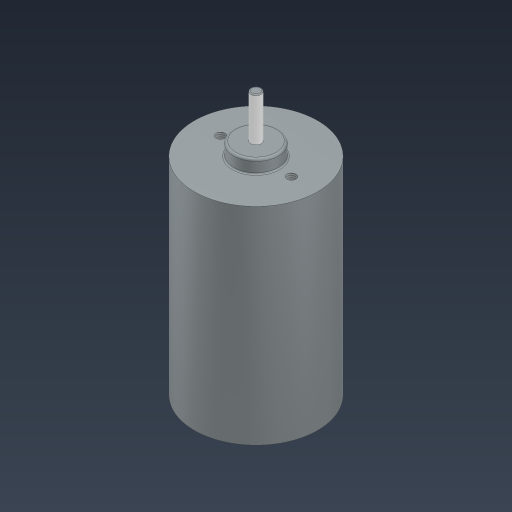
# Autodesk Inventor part: RS395
Saved by Autodesk Inventor 2023 (Build 270158000, 158)
## iProperties
Created: 2025-03-29
Part Number: RS395
Material: Generic
Document SubType Name: Modeling
Designer: szymo
Density: 3.59791 g/cm^3
Appearance: Zinc(1)
Mass: 114.3 g
Surface Area: 60.0998 cm^2
Volume: 31.7685 cm^3
Author: szymo
Autodesk Inventor part; units mm, degrees
ref_plane "YZ Plane" through (0, 0, 0) normal (1, 0, 0) x (0, 1, 0)
ref_plane "XZ Plane" through (0, 0, 0) normal (0, 1, 0) x (-1, 0, 0)
ref_plane "XY Plane" through (0, 0, 0) normal (0, 0, 1) x (1, 0, 0)
sketch "Sketch1" plane through (0, 0, 0) normal (0, 1, 0) x (-1, 0, 0)
  circle A0 centre (0, 0) radius 13.85
  circle A1 centre (0, 0) radius 5
  dimension "d0" = 27.7
  dimension "d3" = 10
  constraints: 2 centre point, 2 coincident
  measures "d0" diameter of A0
  measures "d3" diameter of A1
extrude "Extrusion1" add sketch "Sketch1" along normal blind 46.5 contours A0 | A1
extrude "Extrusion2" add sketch "Sketch1" against normal blind 5.2 contours A1
sketch "Sketch2" plane through (0, 46.5, 0) normal (0, 1, 0) x (1, 0, 0)
  circle A0 centre (0, 0) radius 5
  circle A1 centre (0, 0) radius 1.15
  dimension "d6" = 10
  dimension "d7" = 2.3
  constraints: 2 centre point, 2 coincident
  measures "d6" diameter of A0
  measures "d7" diameter of A1
extrude "Extrusion3" add sketch "Sketch2" along normal blind 3
extrude "Extrusion4" add sketch "Sketch2" along normal blind 12.8 contours A1
ref_plane "Work Plane1" through (0, 41.5, 0) normal (0, 1, 0) x (1, 0, 0)
sketch "Sketch4" plane through (0, 41.5, 0) normal (0, 1, 0) x (1, 0, 0)
  circle A0 centre (0, 0) radius 15.05
  circle A1 centre (0, 0) radius 13.85 projected
  circle A2 centre (0, 0) radius 5 projected
  dimension "d13" = 30.1
  constraints: 1 centre point, 1 coincident
  measures "d13" diameter of A0
extrude "Extrusion5" [suppressed]
sketch "Sketch5" plane through (0, 46.5, 0) normal (0, 1, 0) x (1, 0, 0)
  circle A0 centre (0, 0) radius 1.15 construction
  circle A1 centre (0, 0) radius 6.8 construction
  circle A2 centre (0, 0) radius 13.85 construction
  circle A3 centre (0, 0) radius 9.15 construction
  circle A4 centre (7.975, 0) radius 1.175
  circle A5 centre (-7.975, 0) radius 1.175
  line L0 (0, 0) -> (7.975, 0) construction
  line L1 (0, 0) -> (-7.975, 0) construction
  dimension "d16" = 13.6
  dimension "d17" = 4.7
  constraints: 6 coincident, 4 centre point, 4 end point, 4 tangent, 2 horizontal
  measures "d16" diameter of A1
  measures "d17" radial gap between concentric circles of A2 A3
hole "Hole1" at (-7.975, 46.5, 0) at (7.975, 46.5, 0) direction (0, -1, 0) diameter 2.013 depth 4 thread size "M2.5x0.45" class "6H" standard "ISO Metric profile"
sketch "Sketch6" plane through (0, 0, 0) normal (1, 0, 0) x (0, 1, 0)
  line L0 (-5.2, 5) -> (-5.2, -5) projected
  line L1 (0, -5) -> (0, 5) projected
  line L2 (0, 0) -> (-6.1046, 0)
  line L3 (0, 5) -> (-5.2, 5) projected
  line L4 (-3.3, 5) -> (-3.3, 3.5)
  line L5 (-3.3, 3.5) -> (-4.3, 3.5)
  line L6 (-4.3, 3.5) -> (-4.3, 1.15)
  line L7 (-4.3, 1.15) -> (-5.2, 1.15)
  line L8 (-5.2, 5) -> (-5.2, -5) projected
  point P0 (-5.2, 0)
  dimension "d25" = 0.9
  dimension "d26" = 1.15
  dimension "d27" = 1
  dimension "d28" = 3.5
  constraints: 10 end point, 3 perpendicular, 2 point on line, 1 horizontal, 1 parallel
  measures "d25" distance of L6.end L7.end
  measures "d26" distance between parallel lines of L2 L7
  measures "d27" distance of L4.end L5.end
  measures "d28" distance between parallel lines of L2 L5
revolve "Revolution1" cut sketch "Sketch6" angle 360 about axis through (0, 0, 0) along (0, -1, 0) contours L3 L4 L5 L6 L7 L0
fillet "Fillet1" radius 0.2 1 edges at (0, -5.2, -1.15)
fillet "Fillet3" radius 1 1 edges at (5, 0, 0)
chamfer "Chamfer1" distance 0.4 angle 45 1 edges at (0, -3.3, -3.5)
fillet "Fillet4" radius 0.2 1 edges at (0, -4.3, -3.5)
fillet "Fillet5" radius 0.5 2 edges at (0, -3.3, -3.9) (0, -3.7, -3.5)
fillet "Fillet6" radius 0.2 1 edges at (-1.15, 59.3, 0)
fillet "Fillet7" radius 0.5 1 edges at (-5, 49.5, 0)
fillet "Fillet8" radius 0.3 1 edges at (-5, 46.5, 0)
body "Solid1"
